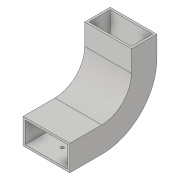
# Autodesk Inventor part: RecTubeNewTapping
Saved by Autodesk Inventor 2018.2 (Build 222227000, 227)
## iProperties
Created: 2018-11-29
Part Number: RecTubeNewTapping
Material: Generic
Document SubType Name: Modeling
Designer: mail
Density: 1 g/cm^3
Appearance: Default
Author: mail
Autodesk Inventor part; units mm, degrees
ref_plane "YZ Plane" through (0, 0, 0) normal (1, 0, 0) x (0, 1, 0)
ref_plane "XZ Plane" through (0, 0, 0) normal (0, 1, 0) x (-1, 0, 0)
ref_plane "XY Plane" through (0, 0, 0) normal (0, 0, 1) x (1, 0, 0)
sketch "Sketch2" plane through (0, 0, 0) normal (0, 0, 1) x (1, 0, 0)
  line L0 (-50, -25) -> (50, -25)
  line L1 (50, -25) -> (50, 25)
  line L2 (50, 25) -> (-50, 25)
  line L3 (-50, 25) -> (-50, -25)
  line L4 (-50, -25) -> (50, 25) construction
  line L5 (50, -25) -> (-50, 25) construction
  line L6 (-55, -30) -> (55, -30)
  line L7 (55, -30) -> (55, 30)
  line L8 (55, 30) -> (-55, 30)
  line L9 (-55, 30) -> (-55, -30)
  line L10 (-55, -30) -> (55, 30) construction
  line L11 (55, -30) -> (-55, 30) construction
  point P0 (0, 0)
  dimension "d0" = 100
  dimension "d1" = 50
  dimension "d2" = 110
  dimension "d3" = 60
  constraints: 24 end point, 4 midpoint, 4 parallel, 2 horizontal, 2 perpendicular
  measures "d0" distance of L2.end L1.end
  measures "d1" distance of L1.end L0.end
  measures "d2" distance of L8.end L7.end
  measures "d3" distance of L7.end L6.end
sketch "Sketch3" plane through (0, 0, 0) normal (1, 0, 0) x (0, 1, 0)
  line L0 (0, 0) -> (0, -75)
  arc A0 (0, -75) -> (100, -175) centre (100, -75) ccw
  line L1 (100, -75) -> (100, -175) construction
  line L2 (100, -75) -> (0, -75) construction
  line L3 (100, -175) -> (150, -175)
  constraints: 8 end point, 2 point on circle, 1 centre point
sweep "Sweep1" add profiles "Sketch2" path "Sketch3"
sketch "Sketch4" plane through (-55, -30, 0) normal (0, -1, 0) x (1, 0, 0)
  circle A0 centre (55, -37.5) radius 3.5
  point P0 (55, 0)
  dimension "d9" = 7
  constraints: 1 centre point
  measures "d9" diameter of A0
extrude "Extrusion1" cut sketch "Sketch4" against normal blind 10
body "Solid1"
